Autodesk Fusion 360 part; units mm, degrees
note: some values were not read from the file. Chosen so that the rebuilt part matches the saved one: which face or edge a step refers to; that a step has no effect; how an offset face is resized.
(part 2 of 2)
extrude "Extrude18" cut sketch "Sketch16" against normal blind 0.5 contours A1 picked at (282.861085, -7.488445) bodies 3
extrude "Extrude19" cut sketch "Sketch16" against normal blind 0.5 contours A2 picked at (284.449858, -101.38478) bodies 3
extrude "Extrude20" cut sketch "Sketch16" against normal blind 0.5 contours A3 picked at (2.311193, -102.112934) bodies 3
fillet "Fillet7" radius 1 4 edges at (292.589975, 95.585788, -9.453789) (288.175761, 95.000001, -9.453789) (283.761548, 94.414215, -9.453789) (283.175761, 51.524398, -9.453789) on bodies 3
fillet "Fillet8" radius 1 4 edges at (4.475846, 51.713536, -9.5) (3.89006, 94.414215, -9.5) (-0.524154, 95.000001, -9.5) (-4.938368, 95.585788, -9.5) on bodies 3
sketch "Sketch3" plane through (293.175761, 0, 0) normal (1, 0, 0) x (0, 1, 0)
  line L0 (-3.89807, 0) -> (104.301737, 0)
  line L1 (104.301737, 0) -> (104.301737, 7.5)
  line L2 (104.301737, 7.5) -> (-3.89807, 7.5)
  line L3 (-3.89807, 7.5) -> (-3.89807, 0)
  line L4 (-3.89807, 0) -> (104.301737, 0)
  line L5 (-3.89807, 0) -> (-3.89807, -7.5)
  line L6 (-3.89807, -7.5) -> (104.301737, -20.029804)
  line L7 (104.301737, 0) -> (104.301737, -20.029804)
  dimension "d5" = 7.5
  constraint horizontal L4
  constraint perpendicular L4 L5
  constraint perpendicular L4 L7
named bodies: "TopCase", "BottomCase", "Plate"
